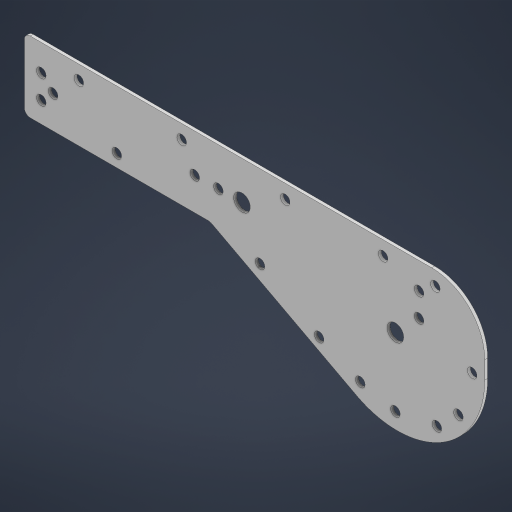
# Autodesk Inventor part: intake sled v5
Saved by Autodesk Inventor 2023.4 (Build 274418000, 418)
## iProperties
Created: 2023-12-16
Part Number: intake sled v5
Material: Generic
Document SubType Name: Modeling
Designer: Meer
Density: 1 g/cm^3
Appearance: Default
Author: Meer
Autodesk Inventor part; units mm, degrees
ref_plane "YZ Plane" through (0, 0, 0) normal (1, 0, 0) x (0, 1, 0)
ref_plane "XZ Plane" through (0, 0, 0) normal (0, 1, 0) x (-1, 0, 0)
ref_plane "XY Plane" through (0, 0, 0) normal (0, 0, 1) x (1, 0, 0)
sketch "Sketch1" plane through (0, 0, 0) normal (0, 0, 1) x (1, 0, 0)
  line L0 (0, 0) -> (247.65, 0)
  line L1 (247.65, 0) -> (247.65, 38.1)
  line L2 (247.65, 38.1) -> (0, 38.1)
  line L3 (0, 38.1) -> (0, 0)
  line L4 (286.1616, 0) -> (255.1962, 0)
  line L5 (255.1962, 0) -> (255.1962, 12.7)
  line L6 (255.1962, 12.7) -> (286.1616, 12.7)
  line L7 (286.1616, 12.7) -> (286.1616, 0)
  line L8 (247.65, 12.7) -> (200.66, 12.7)
  circle A0 centre (200.6294, 0) radius 47.0206
  line L9 (16.2468, 38.1) -> (16.2468, 12.7)
  line L10 (16.2468, 12.7) -> (155.3565, 12.7)
  line L11 (0, 12.7) -> (17.7951, 12.7)
  line L12 (179.5891, -42.0504) -> (75.8552, 12.7)
  point P0 (99.9175, 0)
  dimension "d0" = 247.65
  dimension "d1" = 38.1
  dimension "d2" = 12.7
  dimension "d3" = 30.9654
  dimension "d4" = 46.99
  dimension "d10" = 25.4
  constraints: 26 end point, 7 point on line, 5 perpendicular, 4 parallel, 3 point on circle, 2 horizontal, 1 centre point
  measures "d0" distance of L1.end L2.end
  measures "d1" distance of L0.end L1.end
  measures "d2" distance of L6.end L4.start
  measures "d3" distance of L5.end L6.end
  measures "d4" distance of L8.start L8.end
  measures "d10" distance of L9.start L9.end
extrude "Extrusion1" add sketch "Sketch1" along normal blind 1.5875 contours L3 L11 L10 L12 L0 | L12 L10 A0 L0 | L0 A0 L12 | L3 L2 L9 L11 | A0 L2 L0 | L0 A0 L12 | L10 L9 L2 A0 | A0 L8 L1 | L8 A0 L2 L1
fillet "Fillet1" radius 28.575 1 edges at (247.65, 38.1, 0.7937)
fillet "Fillet2" radius 3.175 1 edges at (0, 38.1, 0.7937)
fillet "Fillet4" radius 3.175 1 edges at (0, 0, 0.7937)
fillet "Fillet5" radius 5.08 1 edges at (99.9175, 0, 0.7937)
sketch "Sketch3" plane through (0, 0, 1.5875) normal (0, 0, 1) x (1, 0, 0)
  line L0 (9.1438, 0) -> (9.1438, 11.176)
  line L1 (9.1438, 11.176) -> (-0.0002, 11.176)
  circle A0 centre (9.1438, 11.176) radius 2.54
  line L2 (9.1438, 11.176) -> (9.1438, 23.876)
  circle A1 centre (9.1438, 23.876) radius 2.54
  line L3 (9.1438, 17.526) -> (15.4938, 17.526)
  circle A2 centre (15.4938, 17.526) radius 2.54
  line L4 (15.4938, 17.526) -> (91.6938, 17.526)
  circle A3 centre (91.6938, 17.526) radius 2.54
  line L5 (91.6938, 17.526) -> (104.3938, 17.526)
  circle A4 centre (104.3938, 17.526) radius 2.54
  line L6 (104.3938, 17.526) -> (117.0938, 17.526)
  circle A5 centre (117.0938, 17.526) radius 4.445
  line L7 (9.1438, 11.176) -> (212.3438, 11.176)
  line L8 (9.1438, 23.876) -> (212.3438, 23.876)
  circle A6 centre (212.3438, 23.876) radius 2.54
  circle A7 centre (212.3438, 11.176) radius 2.54
  line L9 (125.3488, -8.3154) -> (158.5861, -26.9405)
  line L10 (158.5861, -26.9405) -> (180.7442, -39.3573)
  circle A8 centre (29.3464, 30.4847) radius 2.54
  circle A9 centre (84.6567, 30.4847) radius 2.54
  circle A10 centre (140.3584, 30.4847) radius 2.54
  circle A11 centre (192.9921, 30.4847) radius 2.54
  arc A12 (101.0303, -0.5874) -> (98.6591, 0) centre (98.6591, -5.08) ccw projected
  line L11 (98.6591, 0) -> (199.6241, 0)
  line L12 (199.6241, 0) -> (199.6241, -1.778)
  circle A13 centre (199.6241, -1.778) radius 4.445
  line L13 (219.075, 38.1) -> (3.175, 38.1) projected
  line L14 (140.3584, 38.1) -> (140.3584, 30.4847)
  line L15 (192.9921, 38.1) -> (192.9921, 30.4847)
  line L16 (84.6567, 38.1) -> (84.6567, 30.4847)
  line L17 (29.3464, 38.1) -> (29.3464, 30.4847)
  line L18 (221.0918, 31.9182) -> (221.0918, 30.4847)
  circle A14 centre (221.0918, 30.4847) radius 2.54
  line L19 (158.5861, -26.9405) -> (158.5861, -24.4005)
  circle A15 centre (158.5861, -24.4005) radius 2.54
  arc A16 (156.3864, -25.6705) -> (156.3703, -25.6989) centre (158.5861, -26.9405) ccw
  line L20 (180.7442, -39.3573) -> (180.7442, -34.2773)
  circle A17 centre (180.7442, -34.2773) radius 2.54
  line L21 (199.6056, -43.6188) -> (199.6056, -38.5388)
  circle A18 centre (199.6056, -38.5388) radius 2.54
  line L22 (223.6318, -36.189) -> (221.9594, -34.2773)
  circle A19 centre (221.9594, -34.2773) radius 2.54
  line L23 (235.2038, -25.0926) -> (233.5314, -23.1809)
  circle A20 centre (233.5314, -23.1809) radius 2.54
  line L24 (243.4585, 0) -> (240.9185, 0)
  circle A21 centre (240.9185, 0) radius 2.54
  line L25 (125.3488, -8.3154) -> (126.7888, -6.223)
  circle A22 centre (126.7888, -6.223) radius 2.54
  line L26 (49.7674, 4.225) -> (49.7674, 6.765)
  circle A23 centre (49.7674, 6.765) radius 2.54
  point P0 (0, 0)
  point P1 (94.2338, 17.526)
  point P2 (89.1538, 17.526)
  point P3 (6.6038, 11.176)
  point P4 (9.1438, 8.636)
  point P5 (18.0338, 17.526)
  point P6 (12.9538, 17.526)
  point P7 (11.6838, 23.876)
  point P8 (9.1438, 21.336)
  point P9 (125.756, -8.5435)
  dimension "d53" = 5.08
  dimension "d14" = 11.176
  dimension "d15" = 9.144
  dimension "d16" = 5.08
  dimension "d17" = 12.7
  dimension "d18" = 5.08
  dimension "d19" = 6.35
  dimension "d20" = 5.08
  dimension "d21" = 76.2
  dimension "d22" = 5.08
  dimension "d23" = 12.7
  dimension "d24" = 5.08
  dimension "d25" = 12.7
  dimension "d26" = 8.89
  dimension "d27" = 203.2
  dimension "d28" = 203.2
  dimension "d29" = 5.08
  dimension "d30" = 5.08
  dimension "d32" = 38.1
  dimension "d34" = 25.4
  dimension "d40" = 5.08
  dimension "d41" = 5.08
  dimension "d42" = 5.08
  dimension "d43" = 5.08
  dimension "d48" = 100.965
  dimension "d50" = 1.778
  dimension "d51" = 8.89
  dimension "d52" = 5.08
  dimension "d54" = 5.08
  dimension "d55" = 5.08
  dimension "d56" = 5.08
  dimension "d57" = 5.08
  dimension "d58" = 5.08
  dimension "d59" = 5.08
  dimension "d60" = 5.08
  dimension "d61" = 5.08
  dimension "d62" = 5.08
  constraints: 52 end point, 25 coincident, 22 centre point, 11 vertical, 7 point on line, 6 horizontal, 2 point on circle, 1 midpoint, 1 perpendicular, 3 other
  measures "d14" distance of L0.start L0.end
  measures "d15" distance of L0.end L1.end
  measures "d16" diameter of A0
  measures "d17" distance of L2.start L2.end
  measures "d18" diameter of A1
  measures "d19" distance of L3.start L3.end
  measures "d20" diameter of A2
  measures "d21" distance of L4.start L4.end
  measures "d22" diameter of A3
  measures "d23" distance of L5.start L5.end
  measures "d24" diameter of A4
  measures "d25" distance of L6.start L6.end
  measures "d26" diameter of A5
  measures "d27" distance of L8.start L8.end
  measures "d28" distance of L2.start L7.end
  measures "d29" diameter of A6
  measures "d30" diameter of A7
  measures "d32" distance of L9.start L9.end
  measures "d34" distance of L10.start L10.end
  measures "d40" diameter of A8
  measures "d41" diameter of A9
  measures "d42" diameter of A10
  measures "d43" diameter of A11
  measures "d48" distance of L11.start L11.end
  measures "d50" distance of L12.start L12.end
  measures "d51" diameter of A13
  measures "d52" diameter of A14
  measures "d54" distance of L20.start L20.end
  measures "d55" diameter of A17
  measures "d56" distance of L21.start L21.end
  measures "d57" diameter of A18
  measures "d58" diameter of A19
  measures "d59" diameter of A20
  measures "d60" diameter of A21
  measures "d61" diameter of A22
  measures "d62" diameter of A23
extrude "Extrusion2" cut sketch "Sketch3" against normal blind 25.4 contours A0 L1 L0 | A6 | A1 L8 L2 | L2 L8 A1 | A5 | A4 L6 L5 | L5 L6 A4 | A3 L5 L4 | L4 L5 A3 | A2 L4 L3 | L3 L4 A2 | A7 | L0 L7 A0 | L1 A0 L2 | L2 A0 L7 | A22 L9 | A17 | A15 L9 | L9 A15 | A8 | A11 | A10 | A9 | A13 | A14 | A18 | A19 | A20 | A21 | A23 picked at (125.3936, -5.8122)
body "Solid1"
